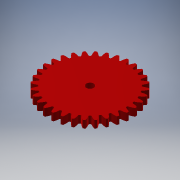
# Autodesk Inventor part: Servo_gear
Saved by Autodesk Inventor 2016 (Build 200138000, 138)
## iProperties
Created: 2015-12-09
Part Number: Servo_gear
Material: Generic
Document SubType Name: Modeling
Designer: lk8187
Density: 1 g/cm^3
Appearance: Smooth - Red
Author: lk8187
Autodesk Inventor part; units mm, degrees
ref_plane "YZ Plane" through (0, 0, 0) normal (1, 0, 0) x (0, 1, 0)
ref_plane "XZ Plane" through (0, 0, 0) normal (0, 1, 0) x (-1, 0, 0)
ref_plane "XY Plane" through (0, 0, 0) normal (0, 0, 1) x (1, 0, 0)
sketch "Sketch1" plane through (0, 0, 0) normal (0, 0, 1) x (1, 0, 0)
  spline S0 degree 3 poles (-1.2962, 16.9505) (-1.2374, 16.8549) (-1.1492, 16.7114) (-1.0407, 16.5147) (-0.9627, 16.3655) (-0.8885, 16.2143) (-0.8186, 16.0611) (-0.7532, 15.9059) (-0.6927, 15.7487) (-0.6379, 15.5894) (-0.5896, 15.4281) (-0.5558, 15.2918) (-0.5336, 15.1818) (-0.5102, 15.1008) (-0.4786, 15.0226) (-0.4372, 14.949) (-0.3933, 14.894) (-0.3536, 14.8542) (-0.3201, 14.8285) (-0.2854, 14.8046) (-0.2475, 14.7862) (-0.2087, 14.7695) (-0.1677, 14.7596) (-0.1264, 14.7512) (-0.0701, 14.7492) (0, 14.7505) (0.0701, 14.7492) (0.1264, 14.7512) (0.1677, 14.7596) (0.2087, 14.7695) (0.2475, 14.7862) (0.2854, 14.8046) (0.3201, 14.8285) (0.3536, 14.8542) (0.3933, 14.894) (0.4372, 14.949) (0.4786, 15.0226) (0.5102, 15.1008) (0.5336, 15.1818) (0.5558, 15.2918) (0.5896, 15.4281) (0.6379, 15.5894) (0.6927, 15.7487) (0.7532, 15.9059) (0.8186, 16.0611) (0.8885, 16.2143) (0.9627, 16.3655) (1.0407, 16.5147) (1.1492, 16.7114) (1.2374, 16.8549) (1.2962, 16.9505) knots 0 0 0 0 0.033676 0.050516 0.067355 0.084194 0.101034 0.117873 0.134712 0.151551 0.168389 0.185227 0.193646 0.202063 0.210481 0.218894 0.227305 0.231514 0.235724 0.239932 0.244142 0.24835 0.25256 0.256768 0.260977 0.269397 0.277817 0.282026 0.286235 0.290444 0.294652 0.298862 0.30307 0.30728 0.311489 0.3199 0.328313 0.336731 0.345149 0.353568 0.370405 0.387244 0.404083 0.420922 0.437761 0.4546 0.471439 0.488279 0.505118 0.538794 0.538794 0.538794 0.538794
  circle A0 centre (0, 0) radius 14.75 construction
  circle A1 centre (0, 0) radius 15.0351 construction
  circle A2 centre (0, 0) radius 16 construction
  circle A3 centre (0, 0) radius 17
  point P0 (-1.1229, 16.6618)
  point P1 (-1.0413, 16.5145)
  point P2 (-0.9633, 16.3652)
  point P3 (-0.8892, 16.214)
  point P4 (-0.8193, 16.0608)
  point P5 (-0.754, 15.9056)
  point P6 (-0.6937, 15.7484)
  point P7 (-0.639, 15.5891)
  point P8 (-0.5909, 15.4277)
  point P9 (-0.5506, 15.2642)
  point P10 (-0.5324, 15.182)
  point P11 (-0.5088, 15.1012)
  point P12 (-0.477, 15.0233)
  point P13 (-0.4353, 14.9502)
  point P14 (-0.383, 14.8844)
  point P15 (-0.353, 14.8549)
  point P16 (-0.3199, 14.8288)
  point P17 (-0.2848, 14.8055)
  point P18 (-0.2473, 14.7865)
  point P19 (-0.2083, 14.7707)
  point P20 (-0.1676, 14.7599)
  point P21 (-0.1262, 14.7524)
  point P22 (-0.0842, 14.75)
  point P23 (0, 14.75)
  point P24 (0.0842, 14.75)
  point P25 (0.1262, 14.7524)
  point P26 (0.1676, 14.7599)
  point P27 (0.2083, 14.7707)
  point P28 (0.2473, 14.7865)
  point P29 (0.2848, 14.8055)
  point P30 (0.3199, 14.8288)
  point P31 (0.353, 14.8549)
  point P32 (0.383, 14.8844)
  point P33 (0.4353, 14.9502)
  point P34 (0.477, 15.0233)
  point P35 (0.5088, 15.1012)
  point P36 (0.5324, 15.182)
  point P37 (0.5506, 15.2642)
  point P38 (0.5909, 15.4277)
  point P39 (0.639, 15.5891)
  point P40 (0.6937, 15.7484)
  point P41 (0.754, 15.9056)
  point P42 (0.8193, 16.0608)
  point P43 (0.8892, 16.214)
  point P44 (0.9633, 16.3652)
  point P45 (1.0413, 16.5145)
  point P46 (1.1229, 16.6618)
  constraints: 4 centre point, 2 point on circle, 103 other
extrude "Extrusion1" add sketch "Sketch1" against normal blind 3
sketch "Sketch2" plane through (0, 0, 0) normal (0, 0, 1) x (1, 0, 0)
  spline S0 degree 3 poles (-0.8725, 9.5113) (-0.8683, 9.5503) (-0.8599, 9.6282) (-0.8392, 9.7439) (-0.8141, 9.8587) (-0.7746, 10.0104) (-0.7157, 10.1973) (-0.6321, 10.417) (-0.5373, 10.6322) (-0.4324, 10.8425) (-0.319, 11.0485) (-0.2364, 11.1817) (-0.1952, 11.2483) knots 0 0 0 0 0.01175 0.0235 0.035251 0.047002 0.070502 0.094002 0.117503 0.141004 0.164506 0.188007 0.188007 0.188007 0.188007
  spline S1 degree 3 poles (0.8725, 9.5113) (0.8683, 9.5503) (0.8599, 9.6282) (0.8392, 9.7439) (0.8141, 9.8587) (0.7746, 10.0104) (0.7157, 10.1973) (0.6321, 10.417) (0.5373, 10.6322) (0.4324, 10.8425) (0.319, 11.0485) (0.2364, 11.1817) (0.1952, 11.2483) knots 0 0 0 0 0.01175 0.0235 0.035251 0.047002 0.070502 0.094002 0.117503 0.141004 0.164506 0.188007 0.188007 0.188007 0.188007
  circle A0 centre (0, 0) radius 11.25 construction
  circle A1 centre (0, 0) radius 9.3969 construction
  circle A2 centre (0, 0) radius 10 construction
  circle A3 centre (0, 0) radius 9.5513
  circle A4 centre (0, 0) radius 12.9487
  arc A5 (0.1952, 11.2483) -> (-0.1952, 11.2483) centre (0, 0) ccw
  point P0 (-0.8586, 9.628)
  point P1 (-0.8385, 9.7438)
  point P2 (-0.8133, 9.8586)
  point P3 (-0.7839, 9.9723)
  point P4 (-0.7136, 10.1965)
  point P5 (-0.6302, 10.4163)
  point P6 (-0.5356, 10.6314)
  point P7 (-0.431, 10.8418)
  point P8 (-0.3173, 11.0475)
  point P9 (0.8586, 9.628)
  point P10 (0.8385, 9.7438)
  point P11 (0.8133, 9.8586)
  point P12 (0.7839, 9.9723)
  point P13 (0.7136, 10.1965)
  point P14 (0.6302, 10.4163)
  point P15 (0.5356, 10.6314)
  point P16 (0.431, 10.8418)
  point P17 (0.3173, 11.0475)
  constraints: 6 centre point, 6 point on circle, 51 other
extrude "Extrusion2" cut sketch "Sketch1" against normal blind 10 contours A3 S0 picked at (-0.1131, 16.1799)
pattern_circular "Circular Pattern1" count 32 over 360 about axis through (0, 0, 0) along (0, 0, -1) of "Extrusion2"
extrude "Extrusion3" [suppressed]
extrude "Extrusion4" [suppressed]
pattern_circular "Circular Pattern2" [suppressed]
sketch "Sketch3" plane through (0, 0, 0) normal (0, 0, 1) x (1, 0, 0)
  circle A0 centre (0, 0) radius 1.5
  dimension "d14" = 3
  constraints: 1 centre point, 1 coincident
  measures "d14" diameter of A0
extrude "Extrusion5" cut sketch "Sketch3" against normal blind 10
equation "\"Module\" = 1"
equation "\"PressureAngle\" = 20deg"
equation "\"UnitProfileClearance\" = 0.25"
equation "\"UnitRoundRadius\" = 0.35"
equation "\"HeadDiameter\" = 34"
equation "\"RootDiameter\" = 29.5"
equation "\"BaseDiameter\" = 30.07016"
equation "\"PitchDiameter\" = 32"
equation "\"HelixAngle\" = 0"
equation "\"UnitCorrection\" = 0"
equation "\"UnitAddendumModification\" = 0"
equation "\"CircularPitch\" = 3.141593"
equation "\"UnitBacklashShift\" = 0"
equation "\"TotalToolShift\" = 0"
equation "\"IsInternal\" = 0"
body "Solid1"
